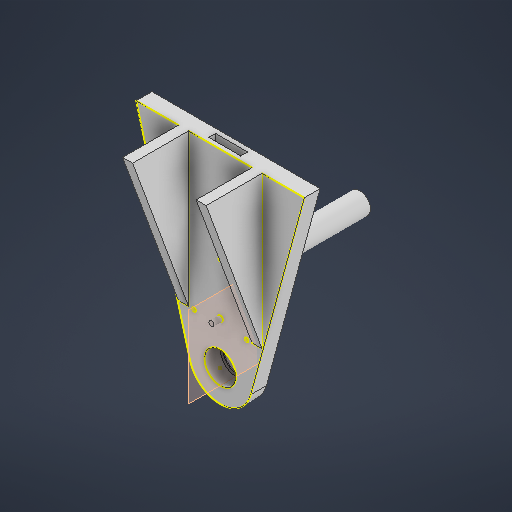
# Autodesk Inventor part: SAFRS-P-0009
Saved by Autodesk Inventor 2026.2 (Build 302298000, 298)
## iProperties
Created: 2025-11-22
Part Number: SAFRS-P-0009
Material: 일반
Document SubType Name: Modeling
Designer: jaewook
Density: 1 g/cm^3
Appearance: 기본값
Author: jaewook
Title: Pitch Axis
Autodesk Inventor part; units mm, degrees
ref_plane "YZ Plane" through (0, 0, 0) normal (1, 0, 0) x (0, 1, 0)
ref_plane "XZ Plane" through (0, 0, 0) normal (0, 1, 0) x (-1, 0, 0)
sketch "스케치1" plane through (0, 0, 0) normal (0, 0, 1) x (1, 0, 0)
  circle A0 centre (0, 0) radius 15
  circle A1 centre (0, 0) radius 30
  line L0 (80, 180) -> (0, 180)
  line L1 (80, 180) -> (28.9502, -7.8668)
  line L2 (-80, 180) -> (0, 180)
  line L3 (-80, 180) -> (-28.9474, -7.8772)
  line L4 (0, 180) -> (0, 141) construction
  circle A2 centre (0, 0) radius 5 projected
  circle A3 centre (0, 0) radius 7.5 projected
  circle A4 centre (0, 0) radius 5.5 projected
  point P0 (-28.9502, -7.8668)
  dimension "d8" = 60
  dimension "d4" = 80
  dimension "d7" = 30
  dimension "d24" = 180
  constraints: 10 end point, 2 coincident, 1 centre point, 1 collinear, 1 horizontal, 1 vertical, 1 vertical alignment, 5 other
  measures "d4" distance of L0.end L0.start
  measures "d7" diameter of A0
  measures "d24" distance from line of L2 A0.centre
extrude "돌출1" add sketch "스케치1" along normal blind 15 contours A1 | A1 L3 L2 L0 L1
sketch "스케치2" plane through (0, 0, 15) normal (0, 0, 1) x (1, 0, 0)
  arc A0 (-28.9502, -7.8668) -> (28.9502, -7.8668) centre (0, 0) ccw projected
  circle A1 centre (0, 0) radius 15 projected
  line L0 (0, 0) -> (0, 40.5)
  line L1 (10, 30.7) -> (-10, 30.7)
  line L2 (-10, 30.7) -> (-10, 85.7)
  line L3 (-10, 85.7) -> (10, 85.7)
  line L4 (10, 85.7) -> (10, 30.7)
  circle A2 centre (0, 40.5) radius 2.45
  dimension "d10" = 9.8
  dimension "d11" = 20
  dimension "d12" = 40.5
  dimension "d13" = 55
  dimension "d14" = 4.9
  constraints: 10 end point, 2 parallel, 1 centre point, 1 coincident, 1 horizontal, 1 perpendicular, 1 vertical, 1 other
  measures "d10" distance from line of L1 L0.end
  measures "d11" distance of L1.start L1.end
  measures "d12" distance of L0.end A0.centre
  measures "d13" distance of L1.end L2.end
  measures "d14" diameter of A2
extrude "돌출2" add sketch "스케치2" along normal blind 8.5 contours A2
sketch "스케치3" plane through (0, 0, 15) normal (0, 0, 1) x (1, 0, 0)
  circle A0 centre (-25, 35.4) radius 2 projected
  circle A1 centre (0, 40.5) radius 2.45 projected
  line L0 (28.9502, -7.8668) -> (80, 180) projected
  line L1 (80, 180) -> (-80, 180) projected
  line L2 (-80, 180) -> (-28.9502, -7.8668) projected
  arc A2 (-28.9502, -7.8668) -> (28.9502, -7.8668) centre (0, 0) ccw projected
  circle A3 centre (0, 0) radius 15 projected
  circle A4 centre (25, 35.4) radius 2 projected
  circle A5 centre (0, 89.2) radius 2 projected
  circle A6 centre (-25, 35.4) radius 1.75
  circle A7 centre (25, 35.4) radius 1.75
  circle A8 centre (0, 89.2) radius 1.75
  dimension "d19" = 3.5
  dimension "d20" = 3.5
  dimension "d21" = 3.5
  constraints: 3 centre point, 3 coincident
  measures "d19" diameter of A6
  measures "d20" diameter of A7
  measures "d21" diameter of A8
extrude "돌출3" cut sketch "스케치3" against normal through all contours A6 | A7 | A8
ref_plane "작업 평면1" through (35, 38.4, 34) normal (1, 0, 0) x (0, 1, 0)
sketch "스케치4" plane through (35, 38.4, 34) normal (1, 0, 0) x (0, 1, 0)
  line L0 (-46.2668, -19) -> (141.6, -19) projected
  line L1 (154.6, -242) -> (154.6, 58) projected
  line L2 (-3, -19) -> (141.6, 34.2157)
  line L3 (-46.2668, -34) -> (141.6, -34) projected
  line L4 (141.6, -34) -> (141.6, -19) projected
  line L5 (-46.2668, -19) -> (141.6, -19) projected
  line L6 (-46.2668, -34) -> (-46.2668, -19) projected
  line L7 (141.6, -19) -> (141.6, 34.2157)
  point P0 (-38.4, -34)
  point P1 (154.6, 58)
  constraints: 4 end point, 1 point on line, 1 vertical, 1 other
extrude "돌출4" add sketch "스케치4" along normal mid plane 9.5 contours L2 L7 L0
mirror "미러1" about plane through (0, 0, 0) normal (1, 0, 0) of "돌출4"
sketch "스케치5" plane through (0, 0, 15) normal (0, 0, 1) x (1, 0, 0)
  line L0 (-39.75, 35.4) -> (-39.75, 180) projected
  line L1 (-39.75, 180) -> (-80, 180) projected
  line L2 (-80, 180) -> (-28.9502, -7.8668) projected
  arc A0 (-28.9502, -7.8668) -> (28.9502, -7.8668) centre (0, 0) ccw projected
  line L3 (28.9502, -7.8668) -> (80, 180) projected
  line L4 (80, 180) -> (39.75, 180) projected
  line L5 (39.75, 180) -> (39.75, 35.4) projected
  line L6 (39.75, 35.4) -> (30.25, 35.4) projected
  line L7 (30.25, 35.4) -> (30.25, 180) projected
  line L8 (30.25, 180) -> (-30.25, 180) projected
  line L9 (-30.25, 180) -> (-30.25, 35.4) projected
  line L10 (-30.25, 35.4) -> (-39.75, 35.4) projected
  circle A1 centre (0, 0) radius 15 projected
  circle A2 centre (0, 40.5) radius 2.45 projected
  circle A3 centre (25, 35.4) radius 1.75 projected
  circle A4 centre (-25, 35.4) radius 1.75 projected
  circle A5 centre (0, 89.2) radius 1.75 projected
sketch "스케치6" plane through (-80, 180, 0) normal (0, 1, 0) x (1, 0, 0)
  line L0 (160, 0) -> (0, 0) projected
  line L1 (110.25, -15) -> (49.75, -15) projected
  line L2 (65, -4.5) -> (95, -4.5)
  line L3 (95, -4.5) -> (95, -10.5)
  line L4 (95, -10.5) -> (65, -10.5)
  line L5 (65, -10.5) -> (65, -4.5)
  line L6 (80, 0) -> (80, -15) construction
  line L7 (64.75, -4.25) -> (95.25, -4.25)
  line L8 (95.25, -4.25) -> (95.25, -10.75)
  line L9 (95.25, -10.75) -> (64.75, -10.75)
  line L10 (64.75, -10.75) -> (64.75, -4.25)
  dimension "d25" = 6
  dimension "d26" = 30
  dimension "d27" = 4.5
  dimension "d28" = 0.25
  constraints: 18 end point, 4 parallel, 3 perpendicular, 1 horizontal, 1 midpoint, 4 other
  measures "d25" distance of L4.end L2.start
  measures "d26" distance of L3.end L4.end
  measures "d27" distance between parallel lines of L0 L2
  measures "d28" distance between parallel lines of L5 L10
extrude "돌출5" cut sketch "스케치6" against normal blind 60.6 contours L2 L3 L4 L5 | L7 L8 L9 L10
sketch "스케치7" plane through (0, 0, 15) normal (0, 0, 1) x (1, 0, 0)
  line L0 (30.25, 180) -> (-30.25, 180) projected
  circle A0 centre (0, 89.2) radius 1.75 projected
  circle A1 centre (0, 130) radius 2
  dimension "d31" = 4
  dimension "d32" = 50
  constraints: 1 centre point, 1 vertical alignment
  measures "d31" diameter of A1
  measures "d32" distance from line of L0 A1.centre
extrude "돌출6" cut sketch "스케치7" against normal through all contours A1
sketch "스케치10" plane through (0, 0, 0) normal (0, 0, -1) x (-1, 0, 0)
  circle A0 centre (0, 0) radius 15 projected
  circle A1 centre (0, 0) radius 12
  circle A2 centre (0, 0) radius 16
  dimension "d42" = 3
  dimension "d43" = 1
  constraints: 2 centre point, 2 coincident
  measures "d42" radial gap between concentric circles of A1 A0
  measures "d43" radial gap between concentric circles of A0 A2
extrude "돌출9" add sketch "스케치10" along normal blind 1 contours A0 | A2
sketch "스케치8" plane through (0, 0, 0) normal (0, 0, -1) x (-1, 0, 0)
  circle A0 centre (0, 89.2) radius 1.75 projected
  circle A1 centre (0, 69.2) radius 10
  dimension "d35" = 20
  dimension "d36" = 20
  constraints: 1 centre point, 1 vertical alignment
  measures "d35" diameter of A1
  measures "d36" distance of A0.centre A1.centre
ref_plane "작업 평면2" through (-80, -30, -118) normal (0, 0, 1) x (1, 0, 0)
extrude "돌출7" add sketch "스케치8" along normal up to surface (118 mm away) separate body contours A1
sketch "스케치9" plane through (0, 69.2, -118) normal (0, 0, -1) x (-1, 0, 0)
  circle A0 centre (0, 0) radius 10 projected
  circle A1 centre (0, 0) radius 1.8
  point P0 (0, -69.2)
  dimension "d39" = 3.6
  constraints: 1 centre point, 1 coincident
  measures "d39" diameter of A1
extrude "돌출8" cut sketch "스케치9" against normal blind 30 contours A1 bodies 2
